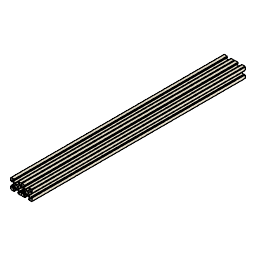
X-Axis Pulley End (Autodesk Fusion 360 archive; units mm, degrees)
design "2040 400mm T-Slot Extrusion"
Autodesk Fusion 360 part; units mm, degrees
sketch "profile" plane through (0, 0, 0) normal (0, 1, 0) x (1, 0, 0)
  circle A0 centre (0, 0) radius 2.5
  line L0 (0, -3.9) -> (-2.5, -3.9)
  line L1 (4, -4) -> (-4, 4) construction
  line L2 (-3.9092, -3.9092) -> (4, 4) construction
  line L3 (10, -10) -> (-10, -10) construction
  line L4 (-10, -10) -> (-10, 10) construction
  line L5 (-10, 10) -> (10, 10) construction
  line L6 (10, 10) -> (10, -10) construction
  line L7 (10, -10) -> (-10, 10) construction
  line L8 (-10, -10) -> (10, 10) construction
  line L9 (8, -8) -> (-8, -8) construction
  line L10 (-8, -8) -> (-8, 8) construction
  line L11 (-8, 8) -> (8, 8) construction
  line L12 (8, 8) -> (8, -8) construction
  line L13 (8, -8) -> (-8, 8) construction
  line L14 (-8, -8) -> (8, 8) construction
  line L15 (0, -8) -> (0, -10) construction
  line L16 (0, -9) -> (-3.1, -9) construction
  line L17 (-3.1, -8) -> (-3.1, -9.6)
  line L18 (-1.75, -10) -> (-1.75, -9.6) construction
  line L19 (0, -9.6) -> (-3.5, -9.6) construction
  line L20 (-3.1, -9.6) -> (-3.5, -9.6)
  line L21 (-3.5, -9.6) -> (-3.5, -10)
  line L22 (0, 0) -> (0, -8) construction
  line L23 (-3.5, -10) -> (-10, -10)
  line L24 (-3.9092, -3.9092) -> (-2.5, -3.9) construction
  line L25 (-8, -8) -> (-6.6, -8) construction
  line L26 (-8, -8) -> (-8, -7) construction
  line L27 (-2.5, -3.9) -> (-6.6, -8)
  line L28 (-6.6, -8) -> (-3.1, -8)
  line L29 (0, -2.5) -> (0, -3.9) construction
  line L30 (-3.9, 0) -> (-3.9, -2.5)
  line L31 (-3.9, -2.5) -> (-8, -6.6)
  line L32 (-8, -6.6) -> (-8, -3.1)
  line L33 (-8, -3.1) -> (-9.6, -3.1)
  line L34 (-9.6, -3.1) -> (-9.6, -3.5)
  line L35 (-9.6, -3.5) -> (-10, -3.5)
  line L36 (-10, -3.5) -> (-10, -10)
  line L37 (0, 0) -> (10, 0) construction
  line L38 (3.9, 0) -> (3.9, -2.5)
  line L39 (3.9, -2.5) -> (8, -6.6)
  line L40 (8, -6.6) -> (8, -3.1)
  line L41 (8, -3.1) -> (9.6, -3.1)
  line L42 (9.6, -3.1) -> (9.6, -3.5)
  line L43 (9.6, -3.5) -> (10, -3.5)
  line L44 (10, -3.5) -> (10, -10)
  line L45 (0, -3.9) -> (2.5, -3.9)
  line L46 (6.6, -8) -> (3.1, -8)
  line L47 (3.1, -8) -> (3.1, -9.6)
  line L48 (3.1, -9.6) -> (3.5, -9.6)
  line L49 (3.5, -9.6) -> (3.5, -10)
  line L50 (3.5, -10) -> (10, -10)
  line L51 (2.5, -3.9) -> (6.6, -8)
  line L52 (-3.9, 0) -> (-3.9, 2.5)
  line L53 (-3.9, 2.5) -> (-8, 6.6)
  line L54 (-8, 6.6) -> (-8, 3.1)
  line L55 (-8, 3.1) -> (-9.6, 3.1)
  line L56 (-9.6, 3.1) -> (-9.6, 3.5)
  line L57 (-9.6, 3.5) -> (-10, 3.5)
  line L58 (-10, 3.5) -> (-10, 10)
  line L59 (0, 3.9) -> (-2.5, 3.9)
  line L60 (-6.6, 8) -> (-3.1, 8)
  line L61 (-3.1, 8) -> (-3.1, 9.6)
  line L62 (-3.1, 9.6) -> (-3.5, 9.6)
  line L63 (-3.5, 9.6) -> (-3.5, 10)
  line L64 (-3.5, 10) -> (-10, 10)
  line L65 (-2.5, 3.9) -> (-6.6, 8)
  line L66 (0, 3.9) -> (2.5, 3.9)
  line L67 (6.6, 8) -> (3.1, 8)
  line L68 (3.1, 8) -> (3.1, 9.6)
  line L69 (3.1, 9.6) -> (3.5, 9.6)
  line L70 (3.5, 9.6) -> (3.5, 10)
  line L71 (3.5, 10) -> (10, 10)
  line L72 (2.5, 3.9) -> (6.6, 8)
  line L73 (3.9, 0) -> (3.9, 2.5)
  line L74 (8, 6.6) -> (8, 3.1)
  line L75 (8, 3.1) -> (9.6, 3.1)
  line L76 (9.6, 3.1) -> (9.6, 3.5)
  line L77 (9.6, 3.5) -> (10, 3.5)
  line L78 (10, 3.5) -> (10, 10)
  line L79 (3.9, 2.5) -> (8, 6.6)
  dimension "d3" = 5
  dimension "d7" = 8
  dimension "d8" = 8
  dimension "d9" = 20
  dimension "d10" = 20
  dimension "d11" = 16
  dimension "d12" = 16
  dimension "d13" = 3.1
  dimension "d14" = 0.4
  dimension "d15" = 3.5
  dimension "d20" = 2.5
  dimension "d21" = 1.4
  constraint coincident A0.centre L22.start
  constraint horizontal L0
  constraint coincident L1 A0.centre
  constraint coincident L2 A0.centre
  constraint horizontal L3
  constraint perpendicular L3 L4
  constraint parallel L3 L5
  constraint parallel L4 L6
  constraint coincident L7 A0.centre
  constraint coincident L8 A0.centre
  constraint horizontal L9
  constraint perpendicular L9 L10
  constraint parallel L9 L11
  constraint parallel L10 L12
  constraint coincident L13 A0.centre
  constraint coincident L14 A0.centre
  constraint midpoint L9 L15.start
  constraint midpoint L3 L15.end
  constraint midpoint L15 L16.start
  constraint perpendicular L15 L16
  constraint coincident L9 L17.start
  constraint perpendicular L3 L17
  constraint coincident L16.end L17
  constraint vertical L18
  constraint coincident L3 L18.start
  constraint coincident L15 L19.start
  constraint perpendicular L15 L19
  constraint coincident L18.end L19
  constraint coincident L19 L17.end
  constraint coincident L3 L21.end
  constraint perpendicular L3 L21
  constraint midpoint L18.end L19
  constraint coincident L9 L25.end
  constraint coincident L10 L26.end
  constraint parallel L14 L27
  constraint coincident L22 L0.start
  constraint coincident L22 L29.start
  constraint coincident A0 L29.start
  constraint parallel L22 L29
  constraint coincident L0.start L29.end
  constraint symmetric L3.end L8 L4.start
  constraint symmetric L8 L17.start L32.end
  constraint symmetric L8 L19.end L34.end
  constraint symmetric L8 L17.end L33.end
  constraint symmetric L8 L21.end L35.end
  constraint symmetric L8 L0.end L30.end
  constraint symmetric L8 L25.end L31.end
  constraint symmetric L8 L0.start L30.start
  constraint midpoint L6 L37.end
  constraint symmetric L3.end L22 L3.start
  constraint symmetric L17.start L22 L46.end
  constraint symmetric L19.end L22 L48.end
  constraint symmetric L17.end L22 L47.end
  constraint symmetric L21.end L22 L49.end
  constraint symmetric L22 L0.end L45.end
  constraint symmetric L22 L25.end L46.start
  constraint symmetric L22 L0.start L29.end
  constraint symmetric L22 L30.start L38.start
  constraint symmetric L22 L30.end L38.end
  constraint symmetric L22 L31.end L39.end
  constraint symmetric L22 L32.end L40.end
  constraint symmetric L22 L33.end L41.end
  constraint symmetric L22 L34.end L42.end
  constraint symmetric L22 L35.end L43.end
  constraint symmetric L22 L3.end L3.start
  constraint symmetric L3.end L37 L4.end
  constraint symmetric L17.start L37 L60.end
  constraint symmetric L19.end L37 L62.end
  constraint symmetric L17.end L37 L61.end
  constraint symmetric L21.end L37 L63.end
  constraint symmetric L0.end L37 L59.end
  constraint symmetric L25.end L37 L60.start
  constraint symmetric L0.start L37 L59.start
  constraint symmetric L30.start L37 L52.start
  constraint symmetric L30.end L37 L52.end
  constraint symmetric L31.end L37 L53.end
  constraint symmetric L32.end L37 L54.end
  constraint symmetric L33.end L37 L55.end
  constraint symmetric L34.end L37 L56.end
  constraint symmetric L35.end L37 L57.end
  constraint symmetric L37 L38.start L73.start
  constraint symmetric L37 L38.end L73.end
  constraint symmetric L37 L39.end L74.start
  constraint symmetric L37 L40.end L74.end
  constraint symmetric L37 L41.end L75.end
  constraint symmetric L37 L42.end L76.end
  constraint symmetric L37 L43.end L77.end
  constraint symmetric L37 L3.start L5.end
  constraint symmetric L37 L0.start L59.start
  constraint symmetric L37 L45.end L66.end
  constraint symmetric L37 L46.start L67.start
  constraint symmetric L37 L46.end L67.end
  constraint symmetric L37 L47.end L68.end
  constraint symmetric L37 L48.end L69.end
  constraint symmetric L37 L49.end L70.end
  measures "d3" diameter of A0
  measures "d7" distance of L1.end L2.end
  measures "d8" distance of L1.start L2.end
  measures "d9" distance of L4.end L5.end
  measures "d10" distance of L3.end L4.end
  measures "d11" distance of L10.end L11.end
  measures "d12" distance of L9.end L10.end
  measures "d13" distance of L16.start L16.end
  measures "d14" distance of L18.start L18.end
  measures "d15" distance of L19.start L19.end
  measures "d20" distance of L0.end L0.start
  measures "d21" distance of L29.start L0.start
extrude "Extrude3" add sketch "profile" along normal blind 400 makes body 1
fillet "Fillet1" radius 0.6 4 edges at (-10, 200, 10) (10, 200, 10) (10, 200, -10) (-10, 200, -10) on bodies 1
fillet "Fillet1" radius 0.2 8 edges at (3.1, 200, 8) (8, 200, 3.1) (8, 200, -3.1) (3.1, 200, -8) (-3.1, 200, 8) (-8, 200, 3.1) (-3.1, 200, -8) (-8, 200, -3.1) on bodies 1
fillet "Fillet1" radius 0.2 8 edges at (-8, 200, 6.6) (-6.6, 200, 8) (6.6, 200, 8) (8, 200, 6.6) (8, 200, -6.6) (6.6, 200, -8) (-6.6, 200, -8) (-8, 200, -6.6) on bodies 1
fillet "Fillet1" radius 0.4 8 edges at (-2.5, 200, 3.9) (2.5, 200, 3.9) (3.9, 200, 2.5) (3.9, 200, -2.5) (2.5, 200, -3.9) (-2.5, 200, -3.9) (-3.9, 200, -2.5) (-3.9, 200, 2.5) on bodies 1
copy_body "CopyPasteBodies1" bodies 1 makes body 2
move_body "Move1" bodies 2 to x (1, 0, 0) y (0, 1, 0) z (0, 0, 1) at (-20, 0, 0)
equation "d13 = ( 6.2 / 2 ) * 1 mm"
equation "d15 = 7 mm / 2"
